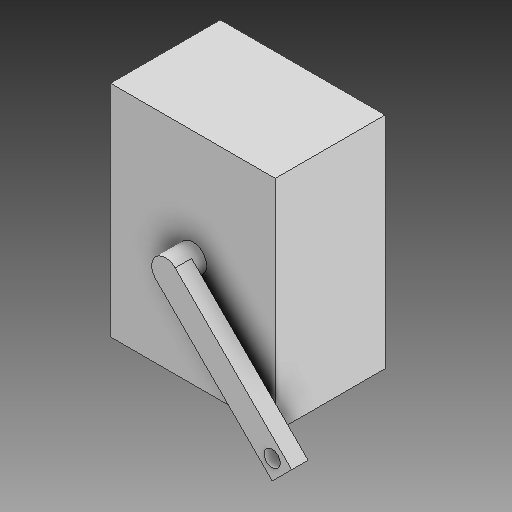
# Autodesk Inventor part: Motor
Saved by Autodesk Inventor 2021 (Build 250183000, 183)
## iProperties
Created: 2022-03-14
Part Number: Motor
Material: Generisch
Document SubType Name: Modeling
Designer: lukas
Density: 1 g/cm^3
Appearance: Vorgabe
Stock Number: Motor
Author: lukas
Autodesk Inventor part; units mm, degrees
ref_plane "YZ Plane" through (0, 0, 0) normal (1, 0, 0) x (0, 1, 0)
ref_plane "XZ Plane" through (0, 0, 0) normal (0, 1, 0) x (-1, 0, 0)
ref_plane "XY Plane" through (0, 0, 0) normal (0, 0, 1) x (1, 0, 0)
sketch "Skizze1" plane through (0, 0, 0) normal (0, 0, 1) x (1, 0, 0)
  line L0 (-21, 0) -> (21, 0) projected
  line L1 (0, -30.3276) -> (0, 25.6724) projected
  line L2 (-15, 17.6724) -> (15, 17.6724)
  line L3 (15, 17.6724) -> (15, -22.3276)
  line L4 (15, -22.3276) -> (-15, -22.3276)
  line L5 (-15, -22.3276) -> (-15, 17.6724)
  point P0 (0, 0)
  dimension "d0" = 40
  dimension "d1" = 30
  constraints: 8 end point, 2 parallel, 1 horizontal, 1 perpendicular
  measures "d0" distance of L4.end L2.start
  measures "d1" distance between parallel lines of L3 L5
extrude "Extrusion1" add sketch "Skizze1" along normal blind 20
sketch "Skizze5" plane through (0, 0, 20) normal (0, 0, 1) x (1, 0, 0)
  circle A0 centre (0, -2.3276) radius 2.5
  line L0 (15, 17.6724) -> (-15, 17.6724) projected
  point P0 (0, 0)
  dimension "d22" = 5
  dimension "d23" = 20
  constraints: 1 centre point
  measures "d22" diameter of A0
  measures "d23" distance from line of L0 A0.centre
extrude "Extrusion5" add sketch "Skizze5" along normal blind 2
sketch "Skizze6" plane through (0, -2.3276, 22) normal (0, 0, 1) x (1, 0, 0)
  circle A0 centre (0, 0) radius 2.5 projected
  line L0 (-2.5, 0) -> (2.5, 0)
  line L1 (1.7678, 1.7678) -> (0, 0)
  line L2 (0, 0) -> (-1.7678, -1.7678)
  line L3 (1.7678, 1.7678) -> (22.981, -19.4454)
  line L4 (22.981, -19.4454) -> (19.4454, -22.981)
  line L5 (19.4454, -22.981) -> (-1.7678, -1.7678)
  circle A1 centre (19.4454, -19.4454) radius 1.4773
  point P0 (0, 2.3276)
  dimension "d26" = 45
  dimension "d27" = 30
  dimension "d28" = 2.5
  dimension "d29" = 2.5
  constraints: 12 end point, 4 point on circle, 2 perpendicular, 1 centre point, 1 horizontal, 1 tangent
  measures "d26" angle of L0 L1
  measures "d27" distance between parallel lines of L4 L2
  measures "d28" distance from line of L3 A1.centre
  measures "d29" distance from line of L4 A1.centre
extrude "Extrusion6" add sketch "Skizze6" along normal blind 3
